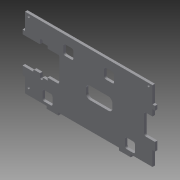
# Autodesk Inventor part: MainPanelCover6
Saved by Autodesk Inventor 2015 (Build 190159000, 159)
## iProperties
Created: 2014-08-06
Part Number: MainPanelCover6
Material: Generic
Document SubType Name: Modeling
Designer: STACKPOLE
Density: 1 g/cm^3
Appearance: Default
Author: STACKPOLE
Autodesk Inventor part; units mm, degrees
ref_plane "YZ Plane" through (0, 0, 0) normal (1, 0, 0) x (0, 1, 0)
ref_plane "XZ Plane" through (0, 0, 0) normal (0, 1, 0) x (-1, 0, 0)
ref_plane "XY Plane" through (0, 0, 0) normal (0, 0, 1) x (1, 0, 0)
sketch "Sketch1" plane through (0, 0, 0) normal (0, 1, 0) x (-1, 0, 0)
  line L0 (153, 85) -> (0, 85)
  line L1 (0, 65) -> (-3, 65)
  line L2 (-3, 65) -> (-3, 60)
  line L3 (-3, 60) -> (0, 60)
  line L4 (0, 40) -> (153, 40) construction
  line L5 (0, 27.5) -> (-3, 27.5)
  line L6 (-3, 27.5) -> (-3, 17.5)
  line L7 (-3, 17.5) -> (0, 17.5)
  line L8 (153, 65) -> (156, 65)
  line L9 (156, 65) -> (156, 60)
  line L10 (156, 60) -> (153, 60)
  line L11 (153, 27.5) -> (156, 27.5)
  line L12 (156, 27.5) -> (156, 17.5)
  line L13 (156, 17.5) -> (153, 17.5)
  line L14 (153, 65) -> (153, 85)
  line L15 (153, 0) -> (153, 17.5)
  line L16 (153, 27.5) -> (153, 60)
  line L17 (0, 85) -> (0, 65)
  line L18 (0, 60) -> (0, 27.5)
  line L19 (0, 17.5) -> (0, 0)
  line L20 (40, 0) -> (40, -3)
  line L21 (40, -3) -> (26, -3)
  line L22 (26, -3) -> (26, 0)
  line L23 (127, 0) -> (127, -3)
  line L24 (127, -3) -> (113, -3)
  line L25 (113, -3) -> (113, 0)
  line L26 (0, 0) -> (26, 0)
  line L27 (40, 0) -> (113, 0)
  line L28 (127, 0) -> (153, 0)
  dimension "d0" = 85
  dimension "d1" = 153
  dimension "d3" = 3
  dimension "d4" = 20
  dimension "d5" = 10
  dimension "d6" = 3
  dimension "d9" = 3
  dimension "d10" = 10
  dimension "d11" = 3
  dimension "d12" = 12.5
  dimension "d13" = 20
  dimension "d16" = 20
  dimension "d39" = 14
  dimension "d40" = 3
  dimension "d41" = 14
  dimension "d42" = 3
  dimension "d43" = 26
  dimension "d44" = 26
  dimension "d64" = 12.5
  dimension "d65" = 5
  dimension "d66" = 5
  constraints: 58 end point, 18 parallel, 13 perpendicular, 9 horizontal, 4 vertical alignment, 2 horizontal alignment, 2 point on line
  measures "d0" distance of L0.end L19.end
  measures "d1" distance of L19.end L15.start
  measures "d3" distance of L1.start L1.end
  measures "d4" distance between parallel lines of L4 L3
  measures "d5" distance of L5.end L6.end
  measures "d6" distance of L6.end L7.end
  measures "d9" distance of L8.start L8.end
  measures "d10" distance of L11.end L12.end
  measures "d11" distance of L12.end L13.end
  measures "d12" distance between parallel lines of L4 L11
  measures "d13" distance between parallel lines of L4 L10
  measures "d16" distance between parallel lines of L0 L1
  measures "d39" distance of L20.end L21.end
  measures "d40" distance of L20.start L20.end
  measures "d41" distance of L23.end L24.end
  measures "d42" distance of L24.end L25.end
  measures "d43" distance between parallel lines of L15 L23
  measures "d44" distance between parallel lines of L19 L22
  measures "d64" distance between parallel lines of L4 L5
  measures "d65" distance of L1.end L2.end
  measures "d66" distance of L8.end L9.end
extrude "Extrusion1" add sketch "Sketch1" along normal blind 3
sketch "Sketch2" plane through (0, 3, 0) normal (0, 1, 0) x (1, 0, 0)
  line L0 (-153, -27.5) -> (-153, -60) projected
  line L1 (0, -60) -> (0, -27.5) projected
  line L2 (-143, -30) -> (-135, -30)
  line L3 (-135, -60) -> (-153, -60)
  line L4 (-135, -24) -> (-132, -24)
  line L5 (-132, -66) -> (-135, -66)
  line L6 (-132, -30) -> (-112, -30)
  line L7 (-112, -30) -> (-112, -60)
  line L8 (-112, -60) -> (-132, -60)
  line L9 (-132, -24) -> (-132, -30)
  line L10 (-132, -60) -> (-132, -66)
  line L11 (-135, -66) -> (-135, -60)
  line L12 (-135, -30) -> (-135, -24)
  line L13 (-153, -60) -> (-153, -30)
  line L14 (3, -27.5) -> (3, -17.5) projected
  line L15 (-153, -40) -> (0, -40) construction
  line L16 (0, -27.5) -> (3, -27.5) projected
  line L17 (-153, -27.5) -> (-143, -27.5)
  line L18 (-143, -27.5) -> (-143, -30)
  point P0 (-156, -60)
  dimension "d22" = 42
  dimension "d24" = 3
  dimension "d26" = 6
  dimension "d29" = 41
  dimension "d67" = 20
  dimension "d68" = 10
  dimension "d69" = 20
  dimension "d70" = 6
  dimension "d109" = 10
  dimension "d154" = 2.5
  constraints: 30 end point, 7 parallel, 4 perpendicular, 4 point on line, 3 horizontal, 2 collinear, 2 vertical alignment, 1 horizontal alignment
  measures "d22" distance between parallel lines of L5 L4
  measures "d24" distance of L4.start L4.end
  measures "d26" distance between parallel lines of L8 L5
  measures "d29" distance between parallel lines of L0 L7
  measures "d67" distance from line of point (-156, -60) L15
  measures "d68" distance between parallel lines of L15 L2
  measures "d69" distance between parallel lines of L3 L15
  measures "d70" distance of L2.end L4.start
  measures "d109" distance of L0.start L17.end
  measures "d154" distance of L17.end L2.start
extrude "Extrusion2" cut sketch "Sketch2" against normal through all
sketch "Sketch3" plane through (0, 3, 0) normal (0, 1, 0) x (1, 0, 0)
  line L0 (-153, -85) -> (0, -85) projected
  line L1 (0, -60) -> (0, -27.5) projected
  line L2 (-112, -30) -> (-112, -60) projected
  line L3 (-48, -37) -> (-48, -42)
  line L4 (-53, -47) -> (-75, -47)
  arc A0 (-48, -37) -> (-53, -32) centre (-53, -37) ccw
  arc A1 (-53, -47) -> (-48, -42) centre (-53, -42) ccw
  arc A2 (-80, -42) -> (-75, -47) centre (-75, -42) ccw
  line L5 (-40, 0) -> (-113, 0) projected
  line L6 (-75, -32) -> (-53, -32)
  line L7 (-80, -42) -> (-80, -37)
  arc A3 (-75, -32) -> (-80, -37) centre (-75, -37) ccw
  point P0 (-115, -26)
  point P1 (-115, -30)
  point P2 (-116, -20)
  point P3 (-79, 0)
  point P4 (-73, 0)
  point P5 (-112, -32)
  point P6 (-112, -26)
  dimension "d34" = 38
  dimension "d35" = 48
  dimension "d116" = 32
  dimension "d117" = 5
  dimension "d177" = 5
  dimension "d178" = 32
  constraints: 8 end point, 8 point on circle, 7 tangent, 4 centre point, 2 equal radius, 2 perpendicular, 2 point on line, 1 horizontal, 1 parallel, 2 other
  measures "d34" distance between parallel lines of L0 L4
  measures "d35" distance between parallel lines of L1 L3
  measures "d116" distance between parallel lines of L5 L6
  measures "d117" radius of A0
  measures "d177" radius of A3
  measures "d178" distance between parallel lines of L7 L3
extrude "Extrusion3" cut sketch "Sketch3" against normal through all
sketch "Sketch6" plane through (0, 0, 0) normal (0, -1, 0) x (1, 0, 0)
  line L0 (0, 27.5) -> (0, 60) projected
  line L1 (-156, 60) -> (-135, 60) projected
  line L2 (0, 52.5) -> (-10, 52.5)
  line L3 (-10, 52.5) -> (-10, 27.5)
  line L4 (-10, 27.5) -> (0, 27.5)
  line L5 (0, 27.5) -> (0, 52.5)
  line L6 (0, 40) -> (-157, 40) construction
  point P0 (-143, 60)
  dimension "d74" = 10
  dimension "d76" = 25
  dimension "d77" = 20
  dimension "d78" = 12.5
  constraints: 10 end point, 2 parallel, 2 perpendicular, 1 horizontal, 1 midpoint, 1 point on line
  measures "d74" distance of L2.start L2.end
  measures "d76" distance of L2.end L3.end
  measures "d77" distance between parallel lines of L1 L6
  measures "d78" distance between parallel lines of L6 L2
extrude "Extrusion6" cut sketch "Sketch6" against normal through all
fillet "Fillet2" radius 2 2 edges at (-10, 1.5, 52.5) (-10, 1.5, 27.5)
fillet "Fillet4" radius 1 1 edges at (-112, 1.5, 60)
sketch "Sketch5" plane through (0, 0, 0) normal (0, -1, 0) x (1, 0, 0)
  line L0 (0, 85) -> (-153, 85) projected
  line L1 (-153, 85) -> (-153, 65) projected
  circle A0 centre (-149, 82) radius 1.5
  circle A1 centre (-149, 8) radius 1.5
  circle A2 centre (-5, 82) radius 1.5
  circle A3 centre (-29, 8) radius 1.5
  point P0 (-154, 50.75)
  dimension "d51" = 3
  dimension "d53" = 4
  dimension "d54" = 3
  dimension "d56" = 3
  dimension "d57" = 74
  dimension "d58" = 144
  dimension "d59" = 3
  dimension "d60" = 3
  dimension "d61" = 24
  constraints: 4 centre point, 2 horizontal alignment, 1 vertical alignment
  measures "d51" diameter of A0
  measures "d53" distance from line of L1 A0.centre
  measures "d54" distance from line of L0 A0.centre
  measures "d56" diameter of A1
  measures "d57" distance of A0.centre A1.centre
  measures "d58" distance of A2.centre A0.centre
  measures "d59" diameter of A2
  measures "d60" diameter of A3
  measures "d61" horizontal distance of A2.centre A3.centre
extrude "Extrusion8" cut sketch "Sketch5" against normal through all
fillet "Fillet10" radius 2 1 edges at (-112, 1.5, 30)
sketch "Sketch10" plane through (0, 0, 0) normal (0, -1, 0) x (1, 0, 0)
  line L0 (-130, 15) -> (-122, 15)
  line L1 (-120, 13) -> (-120, 5)
  line L2 (-122, 3) -> (-130, 3)
  line L3 (-132, 5) -> (-132, 13)
  line L4 (-153, 85) -> (-153, 65) projected
  line L5 (0, 85) -> (-153, 85) projected
  arc A0 (-132, 5) -> (-130, 3) centre (-130, 5) ccw
  arc A1 (-122, 3) -> (-120, 5) centre (-122, 5) ccw
  arc A2 (-120, 13) -> (-122, 15) centre (-122, 13) ccw
  arc A3 (-130, 15) -> (-132, 13) centre (-130, 13) ccw
  line L6 (-31, 15) -> (-23, 15)
  line L7 (-21, 13) -> (-21, 5)
  line L8 (-23, 3) -> (-31, 3)
  line L9 (-33, 5) -> (-33, 13)
  line L10 (0, 65) -> (0, 85) projected
  arc A4 (-31, 15) -> (-33, 13) centre (-31, 13) ccw
  arc A5 (-21, 13) -> (-23, 15) centre (-23, 13) ccw
  arc A6 (-23, 3) -> (-21, 5) centre (-23, 5) ccw
  arc A7 (-33, 5) -> (-31, 3) centre (-31, 5) ccw
  line L11 (-153, 0) -> (-127, 0) projected
  point P0 (0, 0)
  point P1 (-132, 15)
  point P2 (-120, 3)
  point P3 (-132, 3)
  point P4 (-21, 3)
  point P5 (-21, 15)
  point P6 (-33, 3)
  point P7 (-126, 15)
  point P8 (-27, 15)
  dimension "d135" = 12
  dimension "d136" = 12
  dimension "d137" = 21
  dimension "d139" = 2
  dimension "d142" = 12
  dimension "d143" = 12
  dimension "d145" = 21
  dimension "d146" = 2
  dimension "d155" = 3
  constraints: 16 end point, 16 point on circle, 16 tangent, 12 point on line, 8 centre point, 6 equal radius, 4 parallel, 2 horizontal, 2 midpoint, 2 perpendicular, 1 horizontal alignment
  measures "d135" distance of point (-132, 3) point (-132, 15)
  measures "d136" distance of point (-120, 3) point (-132, 3)
  measures "d137" distance between parallel lines of L4 L3
  measures "d139" radius of A0
  measures "d142" distance of point (-21, 3) point (-33, 3)
  measures "d143" distance of point (-21, 15) point (-21, 3)
  measures "d145" distance between parallel lines of L10 L7
  measures "d146" radius of A4
  measures "d155" distance between parallel lines of L11 L2
extrude "Extrusion13" cut sketch "Sketch10" against normal through all
fillet "Fillet11" radius 1 2 edges at (-143, 1.5, 30) (-143, 1.5, 27.5)
fillet "Fillet12" radius 1 2 edges at (-132, 1.5, 66) (-132, 1.5, 24)
fillet "Fillet13" radius 0.5 2 edges at (-135, 1.5, 60) (-135, 1.5, 30)
fillet "Fillet14" radius 1 2 edges at (-135, 1.5, 24) (-135, 1.5, 66)
sketch "Sketch11" plane through (0, 0, 0) normal (0, -1, 0) x (1, 0, 0)
  line L0 (-126, 30) -> (-132, 30)
  line L1 (-132, 30) -> (-132, 27)
  line L2 (-132, 27) -> (-126, 27)
  line L3 (-126, 27) -> (-126, 30)
  line L4 (-114, 30) -> (-132, 30) projected
  line L5 (-132, 30) -> (-132, 25) projected
  line L6 (-132, 60) -> (-126, 60)
  line L7 (-126, 60) -> (-126, 63)
  line L8 (-126, 63) -> (-132, 63)
  line L9 (-132, 63) -> (-132, 60)
  line L10 (-132, 60) -> (-113, 60) projected
  point P0 (0, 0)
  point P1 (-130, 30)
  point P2 (-132, 28)
  point P3 (-130, 60)
  dimension "d158" = 6
  dimension "d159" = 3
  dimension "d163" = 3
  constraints: 16 end point, 4 parallel, 2 horizontal, 2 perpendicular, 2 vertical alignment
  measures "d158" distance of L1.end L2.end
  measures "d159" distance of L2.end L0.start
  measures "d163" distance of L6.end L7.end
extrude "Extrusion14" cut sketch "Sketch11" against normal through all
sketch "Sketch12" plane through (0, 0, 0) normal (0, -1, 0) x (1, 0, 0)
  line L0 (-105, 75) -> (-97, 75)
  line L1 (-95, 73) -> (-95, 65)
  line L2 (-97, 63) -> (-105, 63)
  line L3 (-107, 65) -> (-107, 73)
  line L4 (-107, 75) -> (-95, 63) construction
  line L5 (-95, 75) -> (-107, 63) construction
  line L6 (-153, 85) -> (-153, 65) projected
  line L7 (0, 85) -> (-153, 85) projected
  line L8 (-48, 63) -> (-56, 63)
  line L9 (-58, 65) -> (-58, 73)
  line L10 (-56, 75) -> (-48, 75)
  line L11 (-46, 73) -> (-46, 65)
  line L12 (-46, 63) -> (-58, 75) construction
  line L13 (-58, 63) -> (-46, 75) construction
  line L14 (0, 65) -> (0, 85) projected
  arc A0 (-105, 75) -> (-107, 73) centre (-105, 73) ccw
  arc A1 (-95, 73) -> (-97, 75) centre (-97, 73) ccw
  arc A2 (-97, 63) -> (-95, 65) centre (-97, 65) ccw
  arc A3 (-107, 65) -> (-105, 63) centre (-105, 65) ccw
  arc A4 (-56, 75) -> (-58, 73) centre (-56, 73) ccw
  arc A5 (-46, 73) -> (-48, 75) centre (-48, 73) ccw
  arc A6 (-48, 63) -> (-46, 65) centre (-48, 65) ccw
  arc A7 (-58, 65) -> (-56, 63) centre (-56, 65) ccw
  point P0 (0, 0)
  point P1 (-101, 69)
  point P2 (-52, 69)
  dimension "d166" = 52
  dimension "d167" = 16
  dimension "d168" = 12
  dimension "d169" = 12
  dimension "d170" = 16
  dimension "d171" = 52
  dimension "d172" = 12
  dimension "d173" = 12
  dimension "d174" = 2
  constraints: 24 end point, 16 point on circle, 16 point on line, 16 tangent, 8 centre point, 7 equal radius, 4 midpoint, 4 parallel, 2 horizontal, 2 perpendicular
  measures "d166" distance from line of L6 point (-101, 69)
  measures "d167" distance from line of L7 point (-101, 69)
  measures "d168" distance of L5.end L4.start
  measures "d169" distance of L4.start L5.start
  measures "d170" distance from line of L7 point (-52, 69)
  measures "d171" distance from line of L14 point (-52, 69)
  measures "d172" distance of L13.start L12.end
  measures "d173" distance of L12.end L13.end
  measures "d174" radius of A0
extrude "Extrusion15" cut sketch "Sketch12" against normal through all
body "Solid1"
